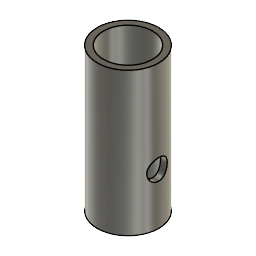
Holder 3 (Autodesk Fusion 360 design; units mm, degrees)
Autodesk Fusion 360 part; units mm, degrees
note: some values were not read from the file. Set by a fixed rule: which sketch regions a step uses.
sketch "Sketch1" plane through (0, 0, 0) normal (0, 0, 1) x (1, 0, 0)
  circle A0 centre (0, 0) radius 15
  circle A1 centre (0, 0) radius 12
  dimension "d1" = 30
  dimension "d2" = -3
  constraint coincident A0.centre A1.centre
  measures "d1" diameter of A0
extrude "Extrude1" add sketch "Sketch1" along normal blind 70
sketch "Sketch2" plane through (0, 0, 0) normal (1, 0, 0) x (0, 1, 0)
  line L0 (0, 0) -> (0, 81)
  circle A0 centre (0, 25) radius 5
  dimension "d5" = 10
  dimension "d6" = 25
  constraint coincident L0.start origin
  constraint vertical L0
  constraint coincident L0 A0.centre
  measures "d5" diameter of A0
  measures "d6" distance of L0.start A0.centre
extrude "Extrude2" cut sketch "Sketch2" along normal through all
